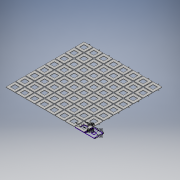
# Autodesk Inventor part: Under Case Button Booster
Saved by Autodesk Inventor 2016 (Build 200138000, 138)
## iProperties
Created: 2016-10-11
Part Number: Under Case Button Booster
Material: Generic
Document SubType Name: Modeling
Designer: Samuel Clay
Density: 1 g/cm^3
Appearance: Default
Author: Samuel Clay
Autodesk Inventor part; units mm, degrees
ref_plane "YZ Plane" through (0, 0, 0) normal (1, 0, 0) x (0, 1, 0)
ref_plane "XZ Plane" through (0, 0, 0) normal (0, 1, 0) x (-1, 0, 0)
ref_plane "XY Plane" through (0, 0, 0) normal (0, 0, 1) x (1, 0, 0)
sketch "Sketch1" plane through (0, 0, 0) normal (0, 1, 0) x (-1, 0, 0)
  line L0 (0, 0) -> (-12.7, 0)
  line L1 (-12.7, 0) -> (-12.7, -12.7)
  line L2 (-12.7, -12.7) -> (0, -12.7)
  line L3 (0, -12.7) -> (0, 0)
  line L4 (-13.97, 0) -> (-26.67, 0)
  line L5 (-26.67, 0) -> (-26.67, -12.7)
  line L6 (-26.67, -12.7) -> (-13.97, -12.7)
  line L7 (-13.97, -12.7) -> (-13.97, 0)
  line L8 (-13.97, -6.6161) -> (-12.7, -6.6161)
  line L9 (-12.7, -6.6161) -> (-12.7, -6.1081)
  line L10 (-12.7, -6.1081) -> (-13.97, -6.1081)
  line L11 (-13.97, -6.1081) -> (-13.97, -6.6161)
  line L12 (-6.35, -12.7) -> (-6.858, -12.7)
  line L13 (-6.858, -12.7) -> (-6.858, -13.97)
  line L14 (-6.858, -13.97) -> (-6.35, -13.97)
  line L15 (-6.35, -13.97) -> (-6.35, -12.7)
  line L16 (-18.415, -4.445) -> (-22.225, -4.445)
  line L17 (-22.225, -4.445) -> (-22.225, -8.255)
  line L18 (-22.225, -8.255) -> (-18.415, -8.255)
  line L19 (-18.415, -8.255) -> (-18.415, -4.445)
  line L20 (-3.175, -3.175) -> (-9.525, -3.175)
  line L21 (-9.525, -3.175) -> (-9.525, -9.525)
  line L22 (-9.525, -9.525) -> (-3.175, -9.525)
  line L23 (-3.175, -9.525) -> (-3.175, -3.175)
  dimension "d0" = 12.7
  dimension "d1" = 12.7
  dimension "d2" = 12.7
  dimension "d3" = 12.7
  dimension "d12" = 0.508
  dimension "d13" = 0.508
  dimension "d14" = 1.27
  dimension "d18" = 1.27
  dimension "d27" = 4.445
  dimension "d28" = 3.175
  constraints: 48 end point, 12 parallel, 6 perpendicular, 4 horizontal, 3 point on line, 1 midpoint, 6 other
  measures "d0" distance of L2.end L1.end
  measures "d1" distance of L1.end L0.end
  measures "d2" distance of L6.end L5.end
  measures "d3" distance of L5.end L4.end
  measures "d12" distance of L10.end L8.start
  measures "d13" distance of L14.end L13.end
  measures "d14" distance between parallel lines of L14 L12
  measures "d18" distance of L8.start L8.end
  measures "d27" distance between parallel lines of L7 L19
  measures "d28" distance between parallel lines of L3 L23
extrude "Extrusion1" add sketch "Sketch1" along normal blind 0.508 contours L3 L2 L1 L0 | L23 L22 L21 L20
extrude "Extrusion2" [suppressed]
feature "FaceDraft2" [suppressed]
extrude "Extrusion4" cut sketch "Sketch1" along normal through all contours L19 L18 L17 L16 | L23 L22 L21 L20
extrude "Extrusion3" add sketch "Sketch1" along normal blind 0.254 draft 50 contours L1 L8 L7 L10 | L15 L14 L13 L2
pattern_linear "Rectangular Pattern2" count 8 spacing 13.97 along (-1, 0, 0) of "Extrusion1", "Extrusion3", "Extrusion4"
pattern_linear "Rectangular Pattern1" count 8 spacing 13.97 along (0, 0, -1) of "Extrusion1", "Extrusion3", "Rectangular Pattern2", "Extrusion4"
body "Solid1"
